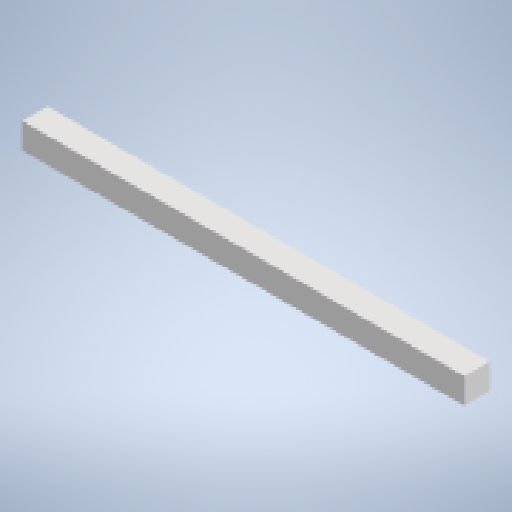
# Autodesk Inventor part: BarraMarco1.1
Saved by Autodesk Inventor 2024 (Build 280153000, 153)
## iProperties
Created: 2023-07-05
Part Number: BarraMarco1.1
Material: Genérico
Document SubType Name: Modeling
Designer: sergi
Density: 1 g/cm^3
Appearance: Valor por defecto
Author: sergi
Autodesk Inventor part; units mm, degrees
ref_plane "YZ Plane" through (0, 0, 0) normal (1, 0, 0) x (0, 1, 0)
ref_plane "XZ Plane" through (0, 0, 0) normal (0, 1, 0) x (-1, 0, 0)
ref_plane "XY Plane" through (0, 0, 0) normal (0, 0, 1) x (1, 0, 0)
sketch "Boceto1" plane through (0, 0, 0) normal (0, 1, 0) x (-1, 0, 0)
  line L0 (-398.2694, -814.4656) -> (-398.2694, 530.5344) projected
  line L1 (-398.2694, 530.5344) -> (122.7306, 530.5344) projected
  line L2 (122.7306, 530.5344) -> (122.7306, -814.4656) projected
  line L3 (122.7306, -814.4656) -> (-398.2694, -814.4656) projected
  line L4 (1000.7306, -844.4656) -> (1000.7306, -1365.4656) projected
  line L5 (1000.7306, -1365.4656) -> (-398.2694, -1365.4656) projected
  line L6 (-398.2694, -1365.4656) -> (-398.2694, -844.4656) projected
  line L7 (-398.2694, -844.4656) -> (1000.7306, -844.4656) projected
  line L8 (1030.7306, -1395.4656) -> (1030.7306, -814.4656) projected
  line L9 (1030.7306, -814.4656) -> (152.7306, -814.4656) projected
  line L10 (152.7306, -814.4656) -> (152.7306, 560.5344) projected
  line L11 (152.7306, 560.5344) -> (-428.2694, 560.5344) projected
  line L12 (-428.2694, 560.5344) -> (-428.2694, -1395.4656) projected
  line L13 (-428.2694, -1395.4656) -> (1030.7306, -1395.4656) projected
  line L14 (-398.2694, 530.5344) -> (-398.2694, 560.5344)
  line L15 (122.7306, 530.5344) -> (122.7306, 560.5344)
  point P0 (0, 0)
  constraints: 4 end point, 2 perpendicular, 2 point on line
extrude "Extrusión1" add sketch "Boceto1" along normal blind 30 contours L14 L11 L15 L1
